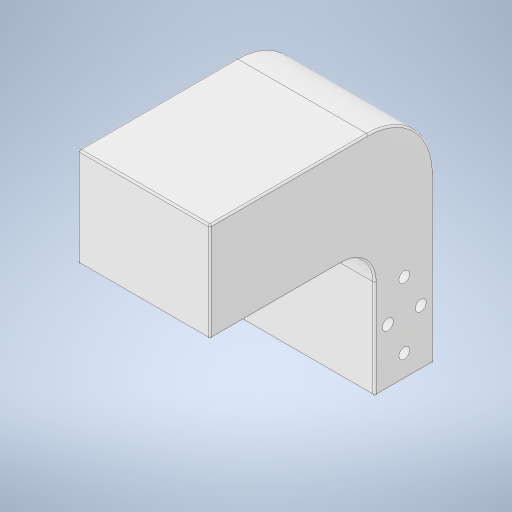
# Autodesk Inventor part: elbow_stopper
Saved by Autodesk Inventor 2024 (Build 280153000, 153)
## iProperties
Created: 2025-06-10
Part Number: elbow_stopper
Material: ABS プラスチック
Document SubType Name: Modeling
Designer: HosodaLab2
Density: 1.06 g/cm^3
Appearance: 滑らか - 白
Author: HosodaLab2
Autodesk Inventor part; units mm, degrees
ref_plane "YZ Plane" through (0, 0, 0) normal (1, 0, 0) x (0, 1, 0)
ref_plane "XZ Plane" through (0, 0, 0) normal (0, 1, 0) x (-1, 0, 0)
ref_plane "XY Plane" through (0, 0, 0) normal (0, 0, 1) x (1, 0, 0)
sketch "スケッチ2" plane through (0, 0, 0) normal (0, 1, 0) x (-1, 0, 0)
  line L0 (-20, 0) -> (-18, 0)
  line L1 (-18, -40) -> (-18, -70)
  line L2 (-18, -70) -> (0, -70)
  line L3 (0, -70) -> (0, -20)
  line L4 (-18, 0) -> (-68, 0)
  line L5 (-68, 0) -> (-68, -30)
  line L6 (-68, -30) -> (-28, -30)
  line L7 (-18, -30) -> (-18, 0)
  arc A0 (0, -20) -> (-20, 0) centre (-20, -20) ccw
  arc A1 (-18, -40) -> (-28, -30) centre (-28, -40) ccw
  point P0 (0, 0)
  point P1 (-38, -10)
  point P2 (-20, 0)
  dimension "d0" = 18
  dimension "d1" = 70
  dimension "d2" = 50
  dimension "d3" = 30
  dimension "d18" = 20
  dimension "d19" = 10
  constraints: 16 end point, 4 parallel, 4 point on circle, 4 point on line, 4 tangent, 2 centre point, 2 horizontal, 2 perpendicular
  measures "d0" distance of L2.end L1.end
  measures "d1" distance of L1.end L0.end
  measures "d2" distance of L7.start L5.end
  measures "d3" distance of L4.end L5.end
  measures "d18" radius of A0
  measures "d19" radius of A1
extrude "押し出し1" add sketch "スケッチ2" along normal blind 40 contours A0 L3 L2 L1 A1 L6 L5 L4
sketch "スケッチ3" plane through (0, 40, 0) normal (0, 1, 0) x (1, 0, 0)
  line L0 (0, 70) -> (0, 0) projected
  line L1 (18, 70) -> (0, 70) projected
  line L2 (14, 53) -> (0, 53) construction
  line L3 (18, 40) -> (18, 70) construction
  line L4 (18, 53) -> (0, 53) construction
  line L5 (9, 70) -> (9, 42.3061) construction
  point P0 (4, 53)
  point P1 (0, 35)
  point P2 (9, 43)
  point P3 (9, 63)
  point P4 (9, 53)
  dimension "d6" = 4
  dimension "d8" = 17
  dimension "d9" = 17
  dimension "d36" = 10
  dimension "d37" = 10
  dimension "d38" = 4
  constraints: 6 end point, 4 point on line, 3 midpoint, 1 collinear, 1 perpendicular, 1 vertical
  measures "d6" horizontal distance of point (4, 53) point (0, 35)
  measures "d8" distance from line of L1 point (4, 53)
  measures "d9" distance from line of L1 L2.start
  measures "d36" distance of point (9, 53) point (9, 43)
  measures "d37" distance of point (9, 63) point (9, 53)
  measures "d38" distance from line of L3 L2.start
hole "穴1" at (4, 40, -53) at (14, 40, -53) at (9, 40, -43) at (9, 40, -63) direction (0, -1, 0) diameter 3.3 end through all
fillet "フィレット1" radius 0.5 14 edges at (48, 40, -30) (68, 40, -15) (0, 40, -45) (18, 40, -55) (9, 40, -70) (18, 20, -70) (18, 0, -55) (48, 0, -30) (68, 20, -30) (68, 20, 0) (68, 0, -15) (0, 0, -45) (9, 0, -70) (0, 20, -70)
sketch "スケッチ5" plane through (0, 40, 0) normal (0, 1, 0) x (1, 0, 0)
  line L0 (17.5, 69.5) -> (0.5, 69.5) projected
  line L1 (67.5, 30) -> (28, 30) projected
  line L2 (17.5, 69.5) -> (27.5, 69.5)
  line L3 (27.5, 69.5) -> (27.5, 30)
  line L4 (27.5, 30) -> (17.5, 30)
  line L5 (17.5, 30) -> (17.5, 69.5)
  line L6 (20.2, 38.7051) -> (20.2, 66.147) construction
  circle A0 centre (14, 53) radius 1.65 construction
  point P0 (0, 0)
  point P1 (20.2, 42.5)
  point P2 (20.2, 63.5)
  dimension "d20" = 6.2
  dimension "d21" = 10
  dimension "d22" = 10.5
  dimension "d23" = 10.5
  constraints: 10 end point, 3 point on line, 2 parallel, 1 horizontal, 1 perpendicular, 1 vertical
  measures "d20" distance from line of L6 A0.centre
  measures "d21" distance between parallel lines of L3 L5
  measures "d22" vertical distance of A0.centre point (20.2, 63.5)
  measures "d23" vertical distance of point (20.2, 42.5) A0.centre
extrude "押し出し2" [suppressed]
sketch "スケッチ6" plane through (0, 40, 0) normal (0, 1, 0) x (1, 0, 0)
  line L0 (20.2, 44.1303) -> (20.2, 62.5) construction
  line L1 (27.5, 62.5) -> (17.5, 62.5) construction
  circle A0 centre (14, 53) radius 1.65 construction
  point P0 (0, 0)
  point P1 (20.2, 42.5)
  point P2 (20.2, 63.5)
  dimension "d26" = 6.2
  dimension "d27" = 10.5
  dimension "d28" = 10.5
  constraints: 3 point on line, 2 end point, 1 vertical
  measures "d26" distance from line of L0 A0.centre
  measures "d27" vertical distance of point (20.2, 63.5) A0.centre
  measures "d28" vertical distance of point (20.2, 42.5) A0.centre
hole "穴2" [suppressed]
